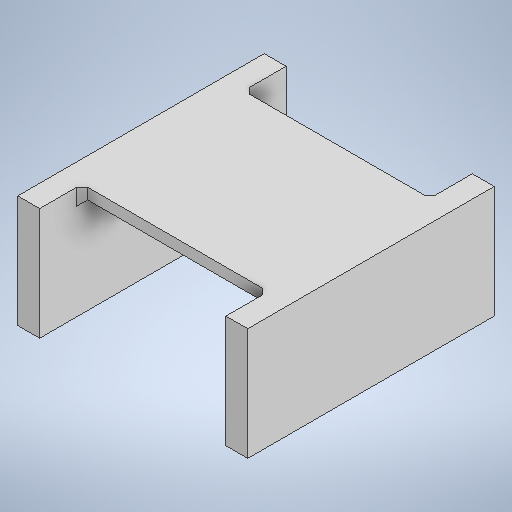
# Autodesk Inventor part: Breadboard_insert
Saved by Autodesk Inventor 2025.2 (Build 292293000, 293)
## iProperties
Created: 2025-09-19
Part Number: Breadboard_insert
Material: Generic
Document SubType Name: Modeling
Designer: TSO
Density: 1 g/cm^3
Appearance: Default
Author: TSO
Autodesk Inventor part; units mm, degrees
ref_plane "YZ Plane" through (0, 0, 0) normal (1, 0, 0) x (0, 1, 0)
ref_plane "XZ Plane" through (0, 0, 0) normal (0, 1, 0) x (-1, 0, 0)
ref_plane "XY Plane" through (0, 0, 0) normal (0, 0, 1) x (1, 0, 0)
sketch "Sketch1" plane through (0, 0, 0) normal (0, 1, 0) x (-1, 0, 0)
  line L0 (0, 0) -> (84, 0)
  line L1 (84, 0) -> (84, -90)
  line L2 (84, -90) -> (0, -90)
  line L3 (0, -90) -> (0, 0)
  line L4 (84, 0) -> (76, 0)
  line L5 (76, 0) -> (8, 0)
  line L6 (8, 0) -> (8, -15.5)
  line L7 (8, -15.5) -> (76, -15.5)
  line L8 (76, -15.5) -> (76, 0)
  line L9 (84, -45) -> (0, -45) construction
  line L10 (8, -90) -> (8, -74.5)
  line L11 (8, -74.5) -> (76, -74.5)
  line L12 (76, -74.5) -> (76, -90)
  dimension "d0" = 84
  dimension "d1" = 90
  dimension "d4" = 8
  dimension "d5" = 68
  dimension "d6" = 15.5
  constraints: 26 end point, 4 parallel, 4 symmetric about line, 2 horizontal, 2 midpoint, 2 perpendicular, 1 point on line
  measures "d0" distance of L1.end L2.end
  measures "d1" distance of L0.end L1.end
  measures "d4" distance of L0.end L4.end
  measures "d5" distance of L7.end L6.end
  measures "d6" distance of L6.end L5.end
extrude "Extrusion1" add sketch "Sketch1" along normal blind 4 contours L0 L6 L7 L8 L1 L2 L12 L11 L10 L3
sketch "Sketch2" plane through (0, 0, 0) normal (0, -1, 0) x (1, 0, 0)
  line L0 (-84, -90) -> (-84, 0) projected
  line L1 (-76, 0) -> (-76, -15.5) projected
  line L2 (-84, -90) -> (-76, -90)
  line L3 (-76, -90) -> (-76, 0)
  line L4 (-76, 0) -> (-84, 0)
  line L5 (-84, 0) -> (-84, -90)
  line L6 (0, 0) -> (-8, 0)
  line L7 (-8, 0) -> (-8, -90)
  line L8 (-8, -90) -> (0, -90)
  line L9 (0, -90) -> (0, 0)
  constraints: 16 end point, 4 parallel, 2 horizontal, 2 perpendicular, 1 point on line
extrude "Extrusion2" add sketch "Sketch2" along normal blind 37
chamfer "Chamfer1" distance 2 angle 45 6 edges at (-76, 0, -45) (-8, 0, -45) (-8, 2, -74.5) (-76, 2, -74.5) (-8, 2, -15.5) (-76, 2, -15.5)
body "Solid1"
